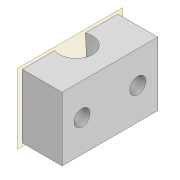
# Autodesk Inventor part: Landing_leg_mount_top
Saved by Autodesk Inventor 2022 (Build 260153000, 153)
## iProperties
Created: 2022-04-29
Part Number: Landing_leg_mount_top
Material: Generic
Document SubType Name: Modeling
Designer: dell
Density: 1 g/cm^3
Appearance: Default
Author: dell
Autodesk Inventor part; units mm, degrees
ref_plane "XZ Plane" through (0, 0, 0) normal (0, 1, 0) x (-1, 0, 0)
ref_plane "XY Plane" through (0, 0, 0) normal (0, 0, 1) x (1, 0, 0)
sketch "Sketch1" plane through (0, 0, 0) normal (0, 1, 0) x (-1, 0, 0)
  circle A0 centre (0, 0) radius 2 construction
  line L0 (5, 6) -> (0, 6)
  line L1 (0, 6) -> (0, -6)
  line L2 (0, -6) -> (5, -6)
  line L3 (5, -6) -> (5, 6)
  line L4 (0, 6) -> (-5, 6)
  line L5 (-5, 6) -> (-5, -6)
  line L6 (-5, -6) -> (0, -6)
  line L7 (0, -6) -> (0, 6)
  dimension "d0" = 4
  dimension "d2" = 5
  dimension "d3" = 6
  dimension "d4" = 6
  dimension "d7" = 5
  constraints: 16 end point, 4 parallel, 2 horizontal, 2 perpendicular, 1 centre point, 1 coincident, 1 collinear, 1 midpoint
  measures "d0" diameter of A0
  measures "d2" distance between parallel lines of L1 L3
  measures "d3" distance from line of point (0, 0) L2
  measures "d4" distance from line of point (0, 0) L0
  measures "d7" distance between parallel lines of L1 L5
extrude "Extrusion1" add sketch "Sketch1" along normal blind 8
ref_plane "Work Plane1" through (5, 8, 6) normal (0.1736482, 0.9848078, 0) x (0, 0, -1)
sketch "Sketch4" plane through (5, 8, 6) normal (0.1736482, 0.9848078, 0) x (0, 0, -1)
  line L0 (6, -3.6708) -> (6, 12.3005) projected
  circle A0 centre (6, 4.2) radius 2.05
  line L1 (0, 0) -> (12, 0) projected
  point P0 (6, 3.5349)
  dimension "d9" = 4.1
  dimension "d12" = 4.2
  constraints: 1 centre point, 1 point on line
  measures "d9" diameter of A0
  measures "d12" distance from line of L1 A0.centre
extrude "Extrusion2" cut sketch "Sketch4" against normal blind 100
sketch "Sketch5" plane through (-5, 0, -6) normal (-1, 0, 0) x (0, 0, 1)
  line L0 (3.95, 8) -> (8.05, 8) projected
  line L1 (8.05, 0) -> (3.95, 0) projected
  circle A0 centre (9.5, 4) radius 1
  circle A1 centre (2.5, 4) radius 1
  line L2 (12, 0) -> (12, 8) projected
  line L3 (0, 0) -> (0, 8) projected
  line L4 (0, 0) -> (12, 0) projected
  point P0 (6, 0)
  dimension "d13" = 2
  dimension "d14" = 2
  dimension "d15" = 2.5
  dimension "d16" = 2.5
  dimension "d17" = 4
  dimension "d18" = 4
  constraints: 2 centre point
  measures "d13" diameter of A0
  measures "d14" diameter of A1
  measures "d15" distance from line of L2 A0.centre
  measures "d16" distance from line of L3 A1.centre
  measures "d17" distance from line of L4 A0.centre
  measures "d18" distance from line of L4 A1.centre
extrude "Extrusion3" cut sketch "Sketch5" against normal blind 100
sketch "Sketch6" plane through (0, 0, 0) normal (1, 0, 0) x (0, 1, 0)
  line L0 (-4.5922, 13.8302) -> (15.486, 13.8302)
  line L1 (15.486, 13.8302) -> (15.486, -16.8326)
  line L2 (15.486, -16.8326) -> (-4.5922, -16.8326)
  line L3 (-4.5922, -16.8326) -> (-4.5922, 13.8302)
  point P0 (0, 0)
  constraints: 8 end point, 2 parallel, 1 horizontal, 1 perpendicular
extrude "Extrusion4" cut sketch "Sketch6" against normal blind 10
equation "\"d4\" = d3"
body "Solid1"
